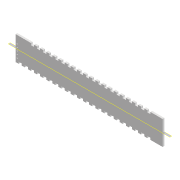
# Autodesk Inventor part: 10_Baseplate_Simmo_side1
Saved by Autodesk Inventor 2022 (Build 260153000, 153)
## iProperties
Created: 2022-08-04
Part Number: 10_Baseplate_Simmo_side1
Material: Generic
Document SubType Name: Modeling
Designer: wanghaoran
Density: 1 g/cm^3
Appearance: Default
Author: wanghaoran
Autodesk Inventor part; units mm, degrees
ref_plane "YZ Plane" through (0, 0, 0) normal (1, 0, 0) x (0, 1, 0)
ref_plane "XZ Plane" through (0, 0, 0) normal (0, 1, 0) x (-1, 0, 0)
ref_plane "XY Plane" through (0, 0, 0) normal (0, 0, 1) x (1, 0, 0)
sketch "Sketch1" plane through (0, 0, 0) normal (0, 0, 1) x (1, 0, 0)
  line L0 (4.9654, 0) -> (4.9654, 6) projected
  line L1 (-450, -9) -> (-450, -67) projected
  line L2 (30, 0) -> (30, 6) projected
  line L3 (30, 6) -> (-450, 6)
  line L4 (-450, 6) -> (-450, -73)
  line L5 (-450, -73) -> (30, -73)
  line L6 (30, -73) -> (30, 6)
  dimension "d26" = 480
  dimension "d27" = 79
  constraints: 8 end point, 2 parallel, 1 horizontal, 1 perpendicular
  measures "d26" distance of L5.end L4.end
  measures "d27" distance of L4.end L3.end
extrude "Extrusion1" add sketch "Sketch1" along normal blind 6
sketch "Sketch2" plane through (0, 0, 6) normal (0, 0, 1) x (1, 0, 0)
  line L0 (-10, 0) -> (-10, 6) projected
  line L1 (-20, 6) -> (-10, 6) projected
  line L2 (-20, 6) -> (-20, 0) projected
  line L3 (-20, 0) -> (-10, 0) projected
  line L4 (-10, 6) -> (-9.9, 6)
  line L5 (-9.9, 6) -> (-9.9, 0)
  line L6 (-9.9, 0) -> (-10, 0)
  line L7 (-10, 0) -> (-10, 6)
  line L8 (-20, 6) -> (-20.1, 6)
  line L9 (-20.1, 6) -> (-20.1, 0)
  line L10 (-20.1, 0) -> (-20, 0)
  line L11 (-20, 0) -> (-20, 6)
  point P0 (0, 0)
  dimension "d5" = 0.1
  dimension "d6" = 0.1
  constraints: 16 end point, 4 parallel, 2 horizontal, 2 perpendicular, 1 point on line
  measures "d5" distance of L5.end L6.end
  measures "d6" distance of L10.end L9.end
extrude "Extrusion2" cut sketch "Sketch2" against normal blind 6
pattern_linear "Rectangular Pattern1" count 20 spacing 20 along (-1, 0, 0) of "Extrusion2"
ref_plane "Work Plane1" through (-450, -33.5, 0) normal (0, -1, 0) x (1, 0, 0)
sketch "Sketch3" plane through (0, 0, 6) normal (0, 0, 1) x (1, 0, 0)
  line L0 (-9.9, 6) -> (-9.9, 0) projected
  line L1 (-20.1, 0) -> (-20.1, 6) projected
  line L2 (126, -33.5) -> (-546, -33.5) projected
  line L3 (-9.9, -73) -> (-9.9, -67)
  line L4 (-20.1, -67) -> (-20.1, -73)
  line L5 (-450, -73) -> (4.9654, -73) projected
  line L6 (-9.9, -67) -> (-20.1, -67)
  point P0 (0, 0)
  constraints: 6 end point, 4 symmetric about line, 1 horizontal
extrude "Extrusion3" cut sketch "Sketch3" against normal blind 6
pattern_linear "Rectangular Pattern2" count 22 spacing 20 along (-1, 0, 0) of "Extrusion3"
sketch "Sketch4" plane through (0, 0, 6) normal (0, 0, 1) x (1, 0, 0)
  circle A0 centre (-445, -59) radius 1.4 projected
  circle A1 centre (-445, -49) radius 1.4 projected
  circle A2 centre (-445, -39) radius 1.4 projected
  circle A3 centre (-445, -29) radius 1.4 projected
  circle A4 centre (-445, -19) radius 1.4 projected
  circle A5 centre (-445, -59) radius 1.6
  line L0 (-445, -59) -> (-445, -49)
  circle A6 centre (-445, -49) radius 1.6
  circle A7 centre (-445, -39) radius 1.6
  circle A8 centre (-445, -29) radius 1.6
  circle A9 centre (-445, -19) radius 1.6
  point P0 (0, 0)
  dimension "d15" = 3.2
  dimension "d18" = 10
  constraints: 5 centre point, 2 end point, 2 vertical, 1 coincident, 8 other
  measures "d15" diameter of A5
  measures "d18" distance of L0.start A6.centre
extrude "Extrusion4" cut sketch "Sketch4" against normal blind 6 contours A0 | A1 | A2 | A3 | A4 | A5 | A6 | A7 | A8 | A9
pattern_linear "Rectangular Pattern3" count 3 spacing 20 along (1, 0, 0) of "Extrusion2"
body "Solid1"
